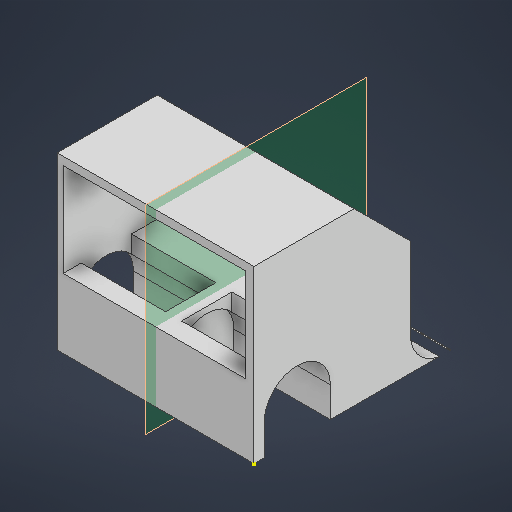
# Autodesk Inventor part: Mini sumô v3
Saved by Autodesk Inventor 2026.1 (Build 301233000, 233)
## iProperties
Created: 2025-11-14
Part Number: Mini sumô v3
Material: Genérico
Document SubType Name: Modeling
Designer: panto
Density: 1 g/cm^3
Appearance: Padrão
Author: panto
Autodesk Inventor part; units mm, degrees
ref_plane "YZ Plane" through (0, 0, 0) normal (1, 0, 0) x (0, 1, 0)
ref_plane "XZ Plane" through (0, 0, 0) normal (0, 1, 0) x (-1, 0, 0)
ref_plane "XY Plane" through (0, 0, 0) normal (0, 0, 1) x (1, 0, 0)
sketch "Esboço1" plane through (0, 0, 0) normal (0, 1, 0) x (-1, 0, 0)
  line L0 (0, 0) -> (98, 0)
  line L1 (98, 0) -> (98, -98)
  line L2 (98, -98) -> (0, -98)
  line L3 (0, -98) -> (0, 0)
  dimension "d0" = 98
  dimension "d1" = 98
  constraints: 8 end point, 2 parallel, 1 horizontal, 1 perpendicular
  measures "d0" distance of L1.end L2.end
  measures "d1" distance of L0.end L1.end
extrude "Extrusão1" add sketch "Esboço1" along normal blind 85
sketch "Esboço2" plane through (0, 0, 0) normal (1, 0, 0) x (0, 0, -1)
  line L0 (98, 0) -> (0, 0) projected
  circle A0 centre (21.5, 15) radius 16.5
  line L1 (38, 15) -> (38, 0)
  line L2 (5, 15) -> (5, 0)
  line L3 (5.2895, 0) -> (38, 0)
  line L4 (98, 85) -> (0, 85) projected
  line L5 (98, 0) -> (98, 85)
  line L6 (53, 85) -> (53, 85)
  line L7 (58, 0) -> (98, 0)
  line L8 (53, 85) -> (98, 85)
  line L9 (98, 85) -> (98, 0)
  line L10 (98, 0) -> (100, 0)
  line L11 (53, 0) -> (53, 85)
  line L12 (98, 0) -> (80, 0)
  line L13 (80, 20) -> (80, 58)
  arc A1 (80, 20) -> (100, 0) centre (100, 20) ccw
  line L14 (80, 58) -> (53, 85)
  line L15 (53, 85) -> (98, 85)
  line L16 (98, 85) -> (98, 0)
  line L17 (98, 0.1003) -> (98, 0)
  point P0 (80, 85)
  point P1 (80, 85)
  dimension "d10" = 33
  dimension "d11" = 45
  dimension "d12" = 18
  dimension "d13" = 20
  dimension "d14" = 27
  dimension "d15" = 27
  constraints: 32 end point, 13 point on line, 8 perpendicular, 5 point on circle, 4 tangent, 2 centre point, 2 collinear, 2 parallel, 1 horizontal, 1 vertical
  measures "d10" diameter of A0
  measures "d11" distance of L4.start L6.end
  measures "d12" distance of L0.start L12.end
  measures "d13" radius of A1
  measures "d14" distance of L13.end point (80, 85)
  measures "d15" distance of L6.start point (80, 85)
extrude "Extrusão2" cut sketch "Esboço2" against normal blind 48 contours L0 A0 L1 | L0 A0 | L0 L2 A0 picked at (26.8574, 18.8676)
extrude "Extrusão3" cut sketch "Esboço2" against normal blind 98 contours A1 L13 L14 L4 L5
sketch "Esboço3" plane through (0, 0, 0) normal (1, 0, 0) x (0, 0, -1)
  line L0 (53, 85) -> (80, 58) projected
  line L1 (53, 85) -> (0, 85) projected
  line L2 (52.5769, 82.2934) -> (77.9758, 56.8945)
  line L3 (77.9758, 56.8945) -> (77.9758, 18.8945)
  line L4 (80, 58) -> (80, 20) projected
  line L5 (98, 0) -> (98, 0.1003) projected
  arc A0 (77.9758, 18.8945) -> (98, 0.1003) centre (94.847, 16.8053) ccw
  line L6 (52.5769, 82.2934) -> (49.7979, 85)
  line L7 (49.7979, 85) -> (53, 85)
  line L8 (49.7979, 85) -> (53, 85)
  line L9 (53, 85) -> (80, 58)
  line L10 (80, 58) -> (80, 20)
  arc A1 (80, 20) -> (98, 0.1003) centre (100, 20) ccw projected
  arc A2 (80, 20) -> (98, 0.1003) centre (100, 20) ccw
  point P0 (0, 0)
  dimension "d21" = 17
  constraints: 14 end point, 4 point on circle, 2 centre point, 2 collinear, 2 parallel, 1 point on line
  measures "d21" radius of A0
sketch "Esboço4" plane through (-98, 0, -98) normal (-1, 0, 0) x (0, 0, 1)
  arc A0 (93, 15) -> (60, 15) centre (76.5, 15) ccw projected
  circle A1 centre (76.5, 15) radius 16.5
  line L0 (60, 15) -> (60, 0) projected
  line L1 (60, 15) -> (60, 0)
  line L2 (93, 15) -> (93, 0)
  line L3 (60, 0) -> (93, 0)
  line L4 (0, 0) -> (98, 0) projected
  constraints: 6 end point, 2 collinear, 1 centre point, 1 coincident, 1 tangent, 1 vertical
extrude "Extrusão4" cut sketch "Esboço4" against normal blind 48 contours A1 L3 A0 | L2 L3 A1 | A1 L3 L0
sketch "Esboço5" plane through (-98, 0, 0) normal (0, 0, 1) x (1, 0, 0)
  line L0 (0, 15) -> (0, 31.5) projected
  line L1 (0, 31.5) -> (0, 34.5)
  line L2 (0, 0) -> (0, 85) projected
  line L3 (0, 34.5) -> (4, 34.5)
  line L4 (0, 85) -> (98, 85) projected
  line L5 (0, 85) -> (3, 85)
  line L6 (3, 85) -> (3, 81)
  line L7 (98, 85) -> (95, 85)
  line L8 (95, 85) -> (95, 81)
  line L9 (98, 0) -> (98, 85) projected
  line L10 (98, 34.5) -> (98, 30.5)
  line L11 (98, 34.5) -> (94, 34.5)
  line L12 (3, 81) -> (94, 81)
  line L13 (94, 81) -> (94, 34.5)
  line L14 (94, 34.5) -> (3, 34.5)
  line L15 (3, 34.5) -> (3, 81)
  point P0 (3, 34.5)
  point P1 (4, 34.5)
  dimension "d24" = 3
  dimension "d25" = 4
  dimension "d26" = 3
  dimension "d27" = 4
  dimension "d28" = 3
  dimension "d29" = 4
  constraints: 24 end point, 5 point on line, 3 horizontal, 3 perpendicular, 2 parallel
  measures "d24" distance of L0.end L1.end
  measures "d25" distance of L1.end L3.end
  measures "d26" distance of L2.end L5.end
  measures "d27" distance of L5.end L6.end
  measures "d28" distance of L4.end L7.end
  measures "d29" distance of L7.end L8.end
extrude "Extrusão5" cut sketch "Esboço5" against normal blind 50 contours L15 L12 L13 L14 L3
ref_plane "Plano de trabalho1" through (-49, 0, 0) normal (-1, 0, 0) x (0, 0, 1)
sketch "Esboço6" plane through (-49, 0, 0) normal (-1, 0, 0) x (0, 0, 1)
  line L0 (0, 34.5) -> (-50, 34.5) projected
  line L1 (-50, 34.5) -> (-80, 34.5)
  line L2 (-80, 34.5) -> (-80, 58)
  line L3 (-50, 81) -> (-50, 34.5) projected
  line L4 (-50, 81) -> (-50, 34.5)
  line L5 (-53, 85) -> (-80, 58) projected
  line L6 (-80, 58) -> (-78, 58)
  line L7 (-78, 58) -> (-53.8179, 81)
  line L8 (-53.8179, 81) -> (-50, 81)
  point P0 (0, 0)
  dimension "d34" = 30
  dimension "d49" = 2
  constraints: 12 end point, 1 collinear, 1 horizontal, 1 parallel, 1 vertical
  measures "d34" distance of L0.end L1.end
  measures "d49" distance of L2.end L6.end
extrude "Extrusão6" cut sketch "Esboço6" along normal mid plane 91.5
sketch "Esboço7" plane through (-95, 34.5, 0) normal (0, 1, 0) x (1, 0, 0)
  line L0 (-3, 38) -> (45, 38) projected
  line L1 (-3, 38) -> (0, 38)
  line L2 (0, 34) -> (42, 34)
  line L3 (42, 34) -> (42, 9)
  line L4 (42, 9) -> (0, 9)
  line L5 (0, 9) -> (0, 34)
  line L6 (47, 38) -> (47, 5) projected
  line L7 (50, 34) -> (92, 34)
  line L8 (92, 34) -> (92, 9)
  line L9 (92, 9) -> (50, 9)
  line L10 (50, 9) -> (50, 34)
  point P0 (95, 0)
  dimension "d38" = 3
  dimension "d39" = 4
  dimension "d40" = 42
  dimension "d43" = 42
  dimension "d44" = 25
  constraints: 18 end point, 4 parallel, 2 horizontal, 2 perpendicular, 1 point on line
  measures "d38" distance of L0.start L1.end
  measures "d39" distance of L1.end L2.start
  measures "d40" distance of L3.end L4.end
  measures "d43" distance of L8.end L9.end
  measures "d44" distance of L7.end L8.end
extrude "Extrusão7" cut sketch "Esboço7" against normal blind 10.5
extrude "Extrusão8" cut sketch "Esboço3" against normal blind 98
sketch "Esboço8" plane through (0, 0, 0) normal (1, 0, 0) x (0, 0, -1)
  point P0 (0, 0)
equation "\"d15\" = d14"
